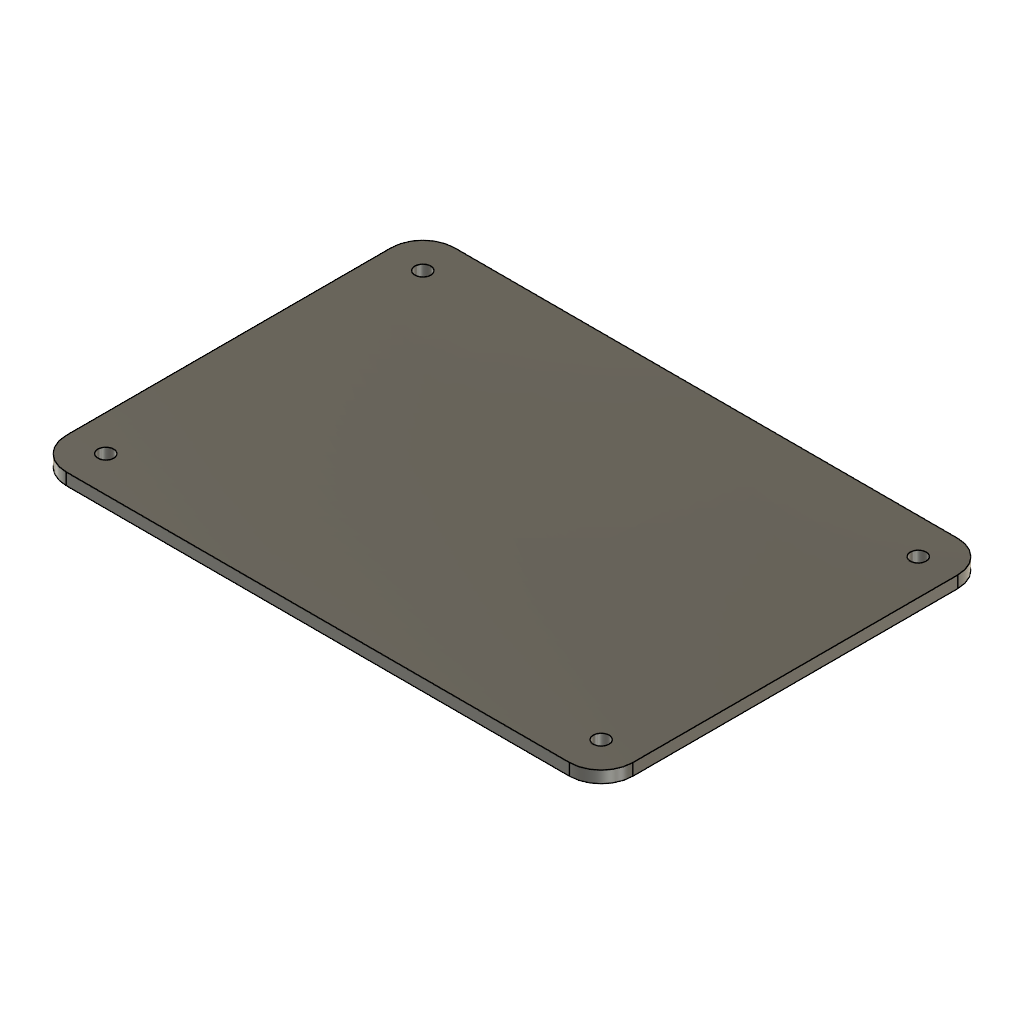
TAPA (Autodesk Fusion 360 design; units mm, degrees)
Autodesk Fusion 360 part; units mm, degrees
sketch "Boceto1" plane through (0, 0, 0) normal (0, 0, 1) x (1, 0, 0)
  line L0 (71.5, 0) -> (-71.5, 0)
  line L1 (0, -49) -> (0, 49)
  line L2 (-71.5, 49) -> (71.5, 49)
  line L3 (71.5, 49) -> (71.5, -49)
  line L4 (71.5, -49) -> (-71.5, -49)
  line L5 (-71.5, -49) -> (-71.5, 49)
  line L6 (-71.5, 49) -> (71.5, -49) construction
  line L7 (71.5, 49) -> (-71.5, -49) construction
  dimension "d1" = 143
  dimension "d2" = 98
  constraint midpoint L0 origin
  constraint horizontal L0
  constraint midpoint L1 origin
  constraint perpendicular L0 L1
  constraint horizontal L2
  constraint perpendicular L2 L3
  constraint parallel L2 L4
  constraint parallel L3 L5
  constraint coincident L6 origin
  constraint coincident L7 origin
  measures "d1" distance of L0.start L0.end
  measures "d2" distance of L1.start L1.end
extrude "Extruir1" add sketch "Boceto1" along normal blind 3
sketch "Boceto2" plane through (0, 0, 3) normal (0, 0, 1) x (-1, 0, 0)
  line L0 (71.5, 49) -> (-71.5, 49)
  line L1 (-71.5, 49) -> (-71.5, -49)
  line L2 (-71.5, -49) -> (71.5, -49)
  line L3 (71.5, -49) -> (71.5, 49)
  line L4 (71.5, -49) -> (62.5, -49)
  line L5 (62.5, -49) -> (62.5, -40)
  line L6 (71.5, 49) -> (62.5, 49)
  line L7 (62.5, 49) -> (62.5, 40)
  line L8 (-71.5, 49) -> (-71.5, 40)
  line L9 (-71.5, 40) -> (-62.5, 40)
  line L10 (-71.5, -49) -> (-62.5, -49)
  line L11 (-62.5, -49) -> (-62.5, -40)
  circle A0 centre (62.5, -40) radius 2
  circle A1 centre (62.5, 40) radius 2
  circle A2 centre (-62.5, -40) radius 2
  circle A3 centre (-62.5, 40) radius 2
  dimension "d7" = 9
  dimension "d8" = 9
  dimension "d9" = 9
  dimension "d10" = 9
  dimension "d11" = 9
  dimension "d12" = 9
  dimension "d13" = 9
  dimension "d14" = 9
  dimension "d15" = 4
  dimension "d16" = 4
  dimension "d17" = 4
  dimension "d18" = 4
  constraint coincident L2.end L3.start
  constraint perpendicular L3 L4
  constraint perpendicular L2 L5
  constraint coincident L0.start L3.end
  constraint perpendicular L3 L6
  constraint perpendicular L6 L7
  constraint coincident L0.end L1.start
  constraint perpendicular L0 L8
  constraint perpendicular L1 L9
  constraint coincident L1.end L2.start
  constraint perpendicular L1 L10
  constraint perpendicular L2 L11
  constraint coincident L5.end A0.centre
  constraint coincident L7.end A1.centre
  constraint coincident L11.end A2.centre
  constraint coincident L9.end A3.centre
  measures "d7" distance of L2.end L4.end
  measures "d8" distance of L4.end L5.end
  measures "d9" distance of L0.start L6.end
  measures "d10" distance of L6.end L7.end
  measures "d11" distance of L0.end L8.end
  measures "d12" distance of L8.end L9.end
  measures "d13" distance of L1.end L10.end
  measures "d14" distance of L10.end L11.end
  measures "d15" diameter of A0
  measures "d16" diameter of A1
  measures "d17" diameter of A2
  measures "d18" diameter of A3
extrude "Extruir2" cut sketch "Boceto2" against normal blind 3 contours A0 | A1 | A2 | A3
fillet "Empalme2" radius 8 4 edges at (-71.5, -49, 1.5) (-71.5, 49, 1.5) (71.5, -49, 1.5) (71.5, 49, 1.5)
